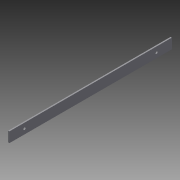
# Autodesk Inventor part: CatchPlate
Saved by Autodesk Inventor 2013 (Build 170138000, 138)
## iProperties
Created: 2014-01-24
Part Number: CatchPlate
Material: Generic
Document SubType Name: Modeling
Designer: Jarod
Density: 1 g/cm^3
Author: Jarod
Autodesk Inventor part; units mm, degrees
ref_plane "YZ Plane" through (0, 0, 0) normal (1, 0, 0) x (0, 1, 0)
ref_plane "XZ Plane" through (0, 0, 0) normal (0, 1, 0) x (-1, 0, 0)
ref_plane "XY Plane" through (0, 0, 0) normal (0, 0, 1) x (1, 0, 0)
sketch "Sketch1" plane through (0, 0, 0) normal (1, 0, 0) x (0, 1, 0)
  line L0 (0, 0) -> (25.4, 0)
  line L1 (25.4, 0) -> (25.4, -406.4)
  line L2 (25.4, -406.4) -> (0, -406.4)
  line L3 (0, -406.4) -> (0, 0)
  dimension "d0" = 25.4
  dimension "d1" = 406.4
  constraints: 8 end point, 2 parallel, 1 horizontal, 1 perpendicular
  measures "d0" distance of L1.end L2.end
  measures "d1" distance of L0.end L1.end
extrude "Extrusion1" add sketch "Sketch1" along normal blind 3.175
sketch "Sketch2" plane through (3.175, 0, 0) normal (1, 0, 0) x (0, 0, -1)
  line L0 (0, 25.4) -> (0, 0) projected
  line L1 (406.4, 0) -> (406.4, 25.4) projected
  line L2 (406.4, 25.4) -> (0, 25.4) projected
  line L3 (0, 12.7) -> (38.1, 12.7)
  line L4 (0, 12.7) -> (38.1, 12.7) construction
  line L5 (406.4, 12.7) -> (368.3, 12.7)
  line L6 (406.4, 12.7) -> (444.5, 12.7) construction
  circle A0 centre (38.1, 12.7) radius 3.175
  circle A1 centre (368.3, 12.7) radius 3.175
  dimension "d4" = 38.1
  dimension "d5" = 0
  dimension "d6" = 38.1
  dimension "d7" = 180
  dimension "d8" = 6.35
  dimension "d9" = 6.35
  constraints: 8 end point, 3 collinear, 2 centre point, 2 coincident, 2 horizontal, 2 midpoint, 1 parallel
  measures "d4" distance of L3.start L3.end
  measures "d5" distance between parallel lines of L3 L4
  measures "d6" distance of L5.start L5.end
  measures "d7" angle of L5 L6
  measures "d8" diameter of A0
  measures "d9" diameter of A1
extrude "Extrusion2" cut sketch "Sketch2" against normal blind 3.175
body "Solid1"
